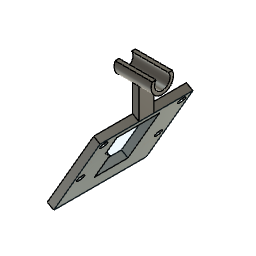
Attache caméra (Autodesk Fusion 360 design; units mm, degrees)
Autodesk Fusion 360 part; units mm, degrees
sketch "Esquisse1" plane through (0, 0, 0) normal (1, 0, 0) x (0, 1, 0)
  circle A0 centre (0, 0) radius 2.1
  circle A1 centre (0, 0) radius 3
  dimension "d1" = 4.2
  dimension "d2" = 6
  constraint coincident A0.centre A1.centre
  constraint concentric A0 A1
  measures "d1" diameter of A0
  measures "d2" diameter of A1
extrude "Extrusion1" add sketch "Esquisse1" along normal blind 10
ref_plane "Plan de construction1" through (5, 0, 0) normal (1, 0, 0) x (0, 1, 0)
sketch "Esquisse3" plane through (0, 0, 0) normal (0, 1, 0) x (1, 0, 0)
  line L0 (4, 0.5) -> (4, 9.5)
  line L1 (4, 9.5) -> (-8.5, 31.1506)
  line L2 (-8.5, 31.1506) -> (-6.7679, 32.1506)
  line L3 (-6.7679, 32.1506) -> (5.7321, 10.5)
  line L4 (5.7321, 10.5) -> (5.7321, 0.5)
  line L5 (4, 9.5) -> (5.7321, 10.5)
  line L6 (4, 0.5) -> (5.7321, 0.5)
  dimension "d7" = 25
  dimension "d8" = 2
  dimension "d9" = 150
  dimension "d47" = 10
  dimension "d52" = 1.7321
  dimension "d53" = 4
  constraint vertical L0
  constraint perpendicular L1 L2
  constraint perpendicular L2 L3
  constraint vertical L4
  constraint perpendicular L1 L5
  constraint perpendicular L4 L6
  measures "d7" distance of L2.end L3.end
  measures "d8" distance of L1.end L2.end
  measures "d9" angle of L0 L1
  measures "d47" distance of L3.end L4.end
  measures "d52" distance of L0 L4
  measures "d53" distance of origin L0
extrude "Extrusion2" add sketch "Esquisse3" along normal blind 2 and the other way blind 2 contours L0 L4 L5 L6
sketch "Esquisse4" plane through (0, -2, 0) normal (0, -1, 0) x (1, 0, 0)
  line L0 (5.7321, -2.2361) -> (4, -2.2361)
  line L1 (4, -2.2361) -> (4, -9.5)
  line L2 (4, -9.5) -> (5.7321, -10.5)
  line L3 (5.7321, -10.5) -> (5.7321, -2.2361)
  line L4 (4, -9.5) -> (-8.5, -31.1506)
  line L5 (-8.5, -31.1506) -> (-6.7679, -32.1506)
  line L6 (-6.7679, -32.1506) -> (5.7321, -10.5)
  dimension "d14" = 150
  dimension "d15" = 25
  dimension "d16" = 2
  constraint coincident L1.end L2.start
  constraint perpendicular L4 L5
  constraint coincident L2.end L3.start
  measures "d14" angle of L1 L4
  measures "d15" distance of L5.end L2.end
  measures "d16" distance of L4.end L5.end
extrude "Extrusion3" add sketch "Esquisse4" along normal blind 10.5 and the other way blind 14.5 contours L2 L4 L5 L6
sketch "Esquisse5" plane through (8.8457, 0, -5.1071) normal (0.866025, 0, -0.5) x (0, 1, 0)
  line L0 (12.5, -6.2272) -> (2, -6.2272)
  line L1 (2, -6.2272) -> (-2, -6.2272)
  line L2 (-2, -6.2272) -> (-12.5, -6.2272)
  line L3 (-12.5, -6.2272) -> (-12.5, -31.2272)
  line L4 (-12.5, -31.2272) -> (12.5, -31.2272)
  line L5 (12.5, -31.2272) -> (12.5, -6.2272)
sketch "Esquisse6" plane through (-0.5179, 0, -21.3253) normal (0.866025, 0, -0.5) x (0, 1, 0)
  circle A0 centre (-10.5, 10.5) radius 1
  circle A1 centre (10.5, 10.5) radius 1
  line L0 (-12.5, 12.5) -> (-12.5, -12.5)
  line L1 (12.5, -12.5) -> (12.5, 12.5)
  line L2 (12.5, 12.5) -> (2, 12.5)
  line L3 (-2, 12.5) -> (-12.5, 12.5)
  circle A2 centre (-10.5, -2) radius 1
  circle A3 centre (10.5, -2) radius 1
  line L4 (-12.5, -12.5) -> (12.5, -12.5)
  line L5 (-4.5, 1.7) -> (4.5, 1.7)
  line L6 (4.5, 1.7) -> (4.5, -6.5)
  line L7 (4.5, -6.5) -> (-4.5, -6.5)
  line L8 (-4.5, -6.5) -> (-4.5, 1.7)
  line L9 (-4.5, 1.7) -> (-7, 4.5)
  line L10 (-7, 4.5) -> (-7, 10.5)
  line L11 (-7, 10.5) -> (4.5, 10.5)
  line L12 (4.5, 10.5) -> (4.5, 1.7)
  dimension "d21" = 21
  dimension "d22" = 2
  dimension "d23" = 2
  dimension "d24" = 2
  dimension "d25" = 2
  dimension "d26" = 2
  dimension "d27" = 2
  dimension "d28" = 21
  dimension "d29" = 12.5
  dimension "d30" = 2
  dimension "d31" = 2
  dimension "d32" = 2
  dimension "d33" = 2
  dimension "d34" = 10.5
  dimension "d35" = 8.2
  dimension "d36" = 9
  dimension "d37" = 8
  dimension "d38" = 6
  dimension "d40" = 8
  dimension "d41" = 11.5
  dimension "d42" = 6
  dimension "d49" = 8
  constraint horizontal L5
  constraint vertical L6
  constraint horizontal L7
  constraint vertical L8
  constraint perpendicular L5 L10
  constraint perpendicular L10 L11
  constraint coincident A1.centre L11
  constraint parallel L6 L12
  measures "d21" distance of A0.centre A1.centre
  measures "d22" distance of A0.centre L0
  measures "d23" distance of A1.centre L1
  measures "d24" distance of A1.centre L2
  measures "d25" distance of A0.centre L3
  measures "d26" diameter of A0
  measures "d27" diameter of A1
  measures "d28" distance of A2.centre A3.centre
  measures "d29" vertical distance of A0.centre A2.centre
  measures "d30" diameter of A2
  measures "d31" diameter of A3
  measures "d32" distance of L1 A3.centre
  measures "d33" distance of L0 A2.centre
  measures "d34" distance of A3.centre L4
  measures "d35" distance of L5.end L6.end
  measures "d36" distance of L5.start L5.end
  measures "d37" distance of L0 L8
  measures "d38" distance of L4 L7
  measures "d40" distance of L1 L12
  measures "d41" distance of L10.end L11.end
  measures "d42" distance of L9.end L10.end
  measures "d49" distance of L1 L6
extrude "Extrusion4" cut sketch "Esquisse6" against normal blind 2
sketch "Esquisse7" plane through (10, 0, 0) normal (1, 0, 0) x (0, 1, 0)
  circle A0 centre (0, 0) radius 2.1
  circle A1 centre (0, 0) radius 3
  line L0 (3.5, 1.25) -> (3.5, 3.5)
  line L1 (3.5, 3.5) -> (-3.5, 3.5)
  line L2 (-3.5, 3.5) -> (-3.5, 1.25)
  arc A2 (-1.6875, 1.25) -> (1.6875, 1.25) centre (0, 0) ccw
  line L3 (-3.5, 1.25) -> (-1.6875, 1.25)
  line L4 (1.6875, 1.25) -> (3.5, 1.25)
  dimension "d54" = 1.25
  constraint concentric A0 A2
  constraint horizontal L3
  constraint vertical L0
  constraint horizontal L1
  constraint vertical L2
  constraint coincident A2.end L3
  constraint collinear L3 L4
  measures "d54" distance of A0.centre L3
extrude "Extrusion5" cut sketch "Esquisse7" against normal blind 10.5 contours A0 A2 | A0 A1 L3 L4 | A1 L0 L1 L2 L3 L4
sketch "Esquisse8" plane through (0, -12.5, 0) normal (0, -1, 0) x (1, 0, 0)
  line L0 (4, -9.5) -> (-8.5, -31.1506)
  line L1 (-8.5, -31.1506) -> (-6.7679, -32.1506)
  line L2 (-6.7679, -32.1506) -> (5.7321, -10.5)
  line L3 (5.7321, -10.5) -> (4, -9.5)
